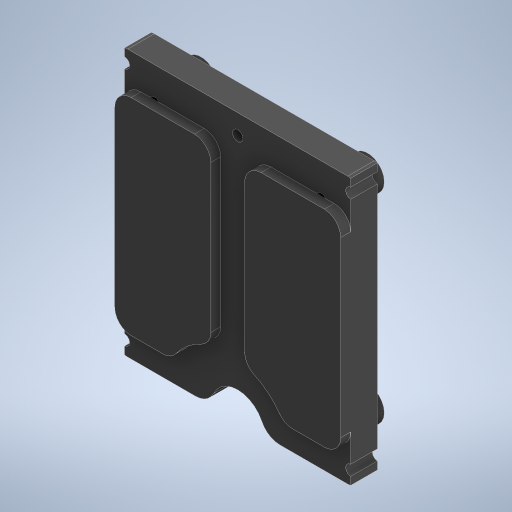
# Autodesk Inventor part: board_cover_inside
Saved by Autodesk Inventor 2024.1 (Build 281209000, 209)
## iProperties
Created: 2024-02-15
Part Number: board_cover_inside
Material: 一般
Document SubType Name: Modeling
Designer: hibik
Density: 1 g/cm^3
Appearance: 既定
Author: hibik
Autodesk Inventor part; units mm, degrees
ref_plane "YZ Plane" through (0, 0, 0) normal (1, 0, 0) x (0, 1, 0)
ref_plane "XZ Plane" through (0, 0, 0) normal (0, 1, 0) x (-1, 0, 0)
ref_plane "XY Plane" through (0, 0, 0) normal (0, 0, 1) x (1, 0, 0)
sketch "スケッチ1" plane through (0, 0, 0) normal (0, 0, 1) x (1, 0, 0)
  line L0 (18.5, 20) -> (-18.5, 20)
  line L1 (-18.5, 20) -> (-18.5, -20)
  line L2 (-18.5, -20) -> (18.5, -20)
  line L3 (18.5, -20) -> (18.5, 20)
  line L4 (18.5, 20) -> (-18.5, -20) construction
  line L5 (-18.5, 20) -> (18.5, -20) construction
  point P0 (0, 0)
  dimension "d0" = 37
  dimension "d1" = 40
  constraints: 12 end point, 2 midpoint, 2 parallel, 1 horizontal, 1 perpendicular
  measures "d0" distance of L2.end L1.end
  measures "d1" distance of L1.end L0.end
extrude "押し出し1" add sketch "スケッチ1" along normal blind 4
sketch "スケッチ3" plane through (0, 0, 4) normal (0, 0, 1) x (1, 0, 0)
  arc A0 (-6.3246, -20) -> (-3.614, -18.2857) centre (-6.3246, -17) ccw projected
  arc A1 (3.614, -18.2857) -> (-3.614, -18.2857) centre (0, -20) ccw projected
  arc A2 (3.614, -18.2857) -> (6.3246, -20) centre (6.3246, -17) ccw projected
  line L0 (19, -20) -> (6.3246, -20) projected
  line L1 (19, -20) -> (19, 20) projected
  line L2 (-19, 20) -> (19, 20) projected
  line L3 (-19, 20) -> (-19, -20) projected
  line L4 (-6.3246, -20) -> (-19, -20) projected
  line L5 (2, -9.0913) -> (2, 13) projected
  arc A3 (5, 16) -> (2, 13) centre (5, 13) ccw projected
  line L6 (5, 16) -> (14.5, 16) projected
  arc A4 (17.5, 13) -> (14.5, 16) centre (14.5, 13) ccw projected
  line L7 (17.5, 13) -> (17.5, -13) projected
  arc A5 (14.5, -16) -> (17.5, -13) centre (14.5, -13) ccw projected
  line L8 (14.5, -16) -> (9.7468, -16) projected
  arc A6 (7.3101, -14.75) -> (9.7468, -16) centre (9.7468, -13) ccw projected
  arc A7 (7.3101, -14.75) -> (3.75, -11.8185) centre (0, -20) ccw projected
  arc A8 (2, -9.0913) -> (3.75, -11.8185) centre (5, -9.0913) ccw projected
  arc A9 (-3.75, -11.8185) -> (-7.3101, -14.75) centre (0, -20) ccw projected
  arc A10 (-9.7468, -16) -> (-7.3101, -14.75) centre (-9.7468, -13) ccw projected
  line L9 (-9.7468, -16) -> (-14.5, -16) projected
  arc A11 (-17.5, -13) -> (-14.5, -16) centre (-14.5, -13) ccw projected
  line L10 (-17.5, -13) -> (-17.5, 13) projected
  arc A12 (-14.5, 16) -> (-17.5, 13) centre (-14.5, 13) ccw projected
  line L11 (-14.5, 16) -> (-5, 16) projected
  arc A13 (-2, 13) -> (-5, 16) centre (-5, 13) ccw projected
  line L12 (-2, 13) -> (-2, -9.0913) projected
  arc A14 (-3.75, -11.8185) -> (-2, -9.0913) centre (-5, -9.0913) ccw projected
  circle A15 centre (-17, -18) radius 0.8 projected
  circle A16 centre (-17, 18) radius 0.8 projected
  circle A17 centre (0, 17) radius 0.8 projected
  circle A18 centre (17, 18) radius 0.8 projected
  circle A19 centre (17, -18) radius 0.8 projected
  point P0 (0, 0)
extrude "押し出し3" add sketch "スケッチ3" along normal blind 1.5 draft -20 contours L5 A3 L6 A4 L7 A5 L8 A6 A7 A8 | A9 A10 L9 A11 L10 A12 L11 A13 L12 A14
fillet "フィレット1" radius 2 4 edges at (-18.5, 20, 2) (18.5, 20, 2) (18.5, -20, 2) (-18.5, -20, 2)
sketch "スケッチ4" plane through (0, 0, 4) normal (0, 0, 1) x (1, 0, 0)
  arc A0 (-6.3246, -20) -> (-3.614, -18.2857) centre (-6.3246, -17) ccw projected
  arc A1 (3.614, -18.2857) -> (-3.614, -18.2857) centre (0, -20) ccw projected
  arc A2 (3.614, -18.2857) -> (6.3246, -20) centre (6.3246, -17) ccw projected
  line L0 (19, -20) -> (6.3246, -20) projected
  line L1 (19, -20) -> (19, 20) projected
  line L2 (-19, 20) -> (19, 20) projected
  line L3 (-19, 20) -> (-19, -20) projected
  line L4 (-6.3246, -20) -> (-19, -20) projected
  line L5 (2, -9.0913) -> (2, 13) projected
  arc A3 (5, 16) -> (2, 13) centre (5, 13) ccw projected
  line L6 (5, 16) -> (14.5, 16) projected
  arc A4 (17.5, 13) -> (14.5, 16) centre (14.5, 13) ccw projected
  line L7 (17.5, 13) -> (17.5, -13) projected
  arc A5 (14.5, -16) -> (17.5, -13) centre (14.5, -13) ccw projected
  line L8 (14.5, -16) -> (9.7468, -16) projected
  arc A6 (7.3101, -14.75) -> (9.7468, -16) centre (9.7468, -13) ccw projected
  arc A7 (7.3101, -14.75) -> (3.75, -11.8185) centre (0, -20) ccw projected
  arc A8 (2, -9.0913) -> (3.75, -11.8185) centre (5, -9.0913) ccw projected
  arc A9 (-3.75, -11.8185) -> (-7.3101, -14.75) centre (0, -20) ccw projected
  arc A10 (-9.7468, -16) -> (-7.3101, -14.75) centre (-9.7468, -13) ccw projected
  line L9 (-9.7468, -16) -> (-14.5, -16) projected
  arc A11 (-17.5, -13) -> (-14.5, -16) centre (-14.5, -13) ccw projected
  line L10 (-17.5, -13) -> (-17.5, 13) projected
  arc A12 (-14.5, 16) -> (-17.5, 13) centre (-14.5, 13) ccw projected
  line L11 (-14.5, 16) -> (-5, 16) projected
  arc A13 (-2, 13) -> (-5, 16) centre (-5, 13) ccw projected
  line L12 (-2, 13) -> (-2, -9.0913) projected
  arc A14 (-3.75, -11.8185) -> (-2, -9.0913) centre (-5, -9.0913) ccw projected
  line L13 (14.5, -16) -> (9.7468, -16) projected
  arc A15 (7.3101, -14.75) -> (9.7468, -16) centre (9.7468, -13) ccw projected
  arc A16 (7.3101, -14.75) -> (3.75, -11.8185) centre (0, -20) ccw projected
  arc A17 (2, -9.0913) -> (3.75, -11.8185) centre (5, -9.0913) ccw projected
  line L14 (2, -9.0913) -> (2, 13) projected
  arc A18 (5, 16) -> (2, 13) centre (5, 13) ccw projected
  line L15 (5, 16) -> (14.5, 16) projected
  arc A19 (17.5, 13) -> (14.5, 16) centre (14.5, 13) ccw projected
  line L16 (17.5, 13) -> (17.5, -13) projected
  arc A20 (14.5, -16) -> (17.5, -13) centre (14.5, -13) ccw projected
  line L17 (-14.5, 16) -> (-5, 16) projected
  arc A21 (-2, 13) -> (-5, 16) centre (-5, 13) ccw projected
  line L18 (-2, 13) -> (-2, -9.0913) projected
  arc A22 (-3.75, -11.8185) -> (-2, -9.0913) centre (-5, -9.0913) ccw projected
  arc A23 (-3.75, -11.8185) -> (-7.3101, -14.75) centre (0, -20) ccw projected
  arc A24 (-9.7468, -16) -> (-7.3101, -14.75) centre (-9.7468, -13) ccw projected
  line L19 (-9.7468, -16) -> (-14.5, -16) projected
  arc A25 (-17.5, -13) -> (-14.5, -16) centre (-14.5, -13) ccw projected
  line L20 (-17.5, -13) -> (-17.5, 13) projected
  arc A26 (-14.5, 16) -> (-17.5, 13) centre (-14.5, 13) ccw projected
  arc A27 (-18.5, -18) -> (-16.5, -20) centre (-16.5, -18) ccw projected
  line L21 (-16.5, -20) -> (16.5, -20) projected
  arc A28 (16.5, -20) -> (18.5, -18) centre (16.5, -18) ccw projected
  line L22 (18.5, -18) -> (18.5, 18) projected
  arc A29 (18.5, 18) -> (16.5, 20) centre (16.5, 18) ccw projected
  line L23 (16.5, 20) -> (-16.5, 20) projected
  arc A30 (-16.5, 20) -> (-18.5, 18) centre (-16.5, 18) ccw projected
  line L24 (-18.5, 18) -> (-18.5, -18) projected
  circle A31 centre (-17, -18) radius 0.8 projected
  circle A32 centre (-17, 18) radius 0.8 projected
  circle A33 centre (0, 17) radius 0.8 projected
  circle A34 centre (17, 18) radius 0.8 projected
  circle A35 centre (17, -18) radius 0.8 projected
  point P0 (0, 0)
  point P1 (-6.3246, -20)
extrude "押し出し4" cut sketch "スケッチ4" against normal through all contours A0 A1 A2 L21
sketch "スケッチ5" plane through (0, 0, 0) normal (0, 0, -1) x (-1, 0, 0)
  circle A0 centre (17, -18) radius 0.8 projected
  circle A1 centre (17, 18) radius 0.8 projected
  circle A2 centre (0, 17) radius 0.8 projected
  circle A3 centre (-17, 18) radius 0.8 projected
  circle A4 centre (-17, -18) radius 0.8 projected
  arc A5 (3.614, -18.2857) -> (6.3246, -20) centre (6.3246, -17) ccw projected
  arc A6 (3.614, -18.2857) -> (-3.614, -18.2857) centre (0, -20) ccw projected
  arc A7 (-6.3246, -20) -> (-3.614, -18.2857) centre (-6.3246, -17) ccw projected
  line L0 (-19, -20) -> (-6.3246, -20) projected
  line L1 (-19, -20) -> (-19, 20) projected
  line L2 (19, 20) -> (-19, 20) projected
  line L3 (19, 20) -> (19, -20) projected
  line L4 (6.3246, -20) -> (19, -20) projected
  line L5 (-2, -9.0913) -> (-2, 13) projected
  arc A8 (-2, 13) -> (-5, 16) centre (-5, 13) ccw projected
  line L6 (-5, 16) -> (-14.5, 16) projected
  arc A9 (-14.5, 16) -> (-17.5, 13) centre (-14.5, 13) ccw projected
  line L7 (-17.5, 13) -> (-17.5, -13) projected
  arc A10 (-17.5, -13) -> (-14.5, -16) centre (-14.5, -13) ccw projected
  line L8 (-14.5, -16) -> (-9.7468, -16) projected
  arc A11 (-9.7468, -16) -> (-7.3101, -14.75) centre (-9.7468, -13) ccw projected
  arc A12 (-3.75, -11.8185) -> (-7.3101, -14.75) centre (0, -20) ccw projected
  arc A13 (-3.75, -11.8185) -> (-2, -9.0913) centre (-5, -9.0913) ccw projected
  arc A14 (7.3101, -14.75) -> (3.75, -11.8185) centre (0, -20) ccw projected
  arc A15 (7.3101, -14.75) -> (9.7468, -16) centre (9.7468, -13) ccw projected
  line L9 (9.7468, -16) -> (14.5, -16) projected
  arc A16 (14.5, -16) -> (17.5, -13) centre (14.5, -13) ccw projected
  line L10 (17.5, -13) -> (17.5, 13) projected
  arc A17 (17.5, 13) -> (14.5, 16) centre (14.5, 13) ccw projected
  line L11 (14.5, 16) -> (5, 16) projected
  arc A18 (5, 16) -> (2, 13) centre (5, 13) ccw projected
  line L12 (2, 13) -> (2, -9.0913) projected
  arc A19 (2, -9.0913) -> (3.75, -11.8185) centre (5, -9.0913) ccw projected
  point P0 (0, 0)
extrude "押し出し5" cut sketch "スケッチ5" against normal through all contours A0 | A1 | A2 | A3 | A4
sketch "スケッチ6" plane through (0, 0, 0) normal (0, 0, -1) x (-1, 0, 0)
  line L0 (-12.5, 15) -> (12.5, 15) construction
  line L1 (12.5, 15) -> (12.5, -15) construction
  line L2 (12.5, -15) -> (-12.5, -15) construction
  line L3 (-12.5, -15) -> (-12.5, 15) construction
  line L4 (-12.5, 15) -> (12.5, -15) construction
  line L5 (12.5, 15) -> (-12.5, -15) construction
  circle A0 centre (-12.5, 15) radius 0.8
  circle A1 centre (12.5, 15) radius 0.8
  circle A2 centre (-12.5, -15) radius 0.8
  circle A3 centre (12.5, -15) radius 0.8
  point P0 (0, 0)
  dimension "d19" = 25
  dimension "d20" = 30
  dimension "d21" = 1.6
  dimension "d22" = 1.6
  dimension "d23" = 1.6
  dimension "d24" = 1.6
  constraints: 12 end point, 4 centre point, 4 coincident, 2 midpoint, 2 parallel, 1 horizontal, 1 perpendicular
  measures "d19" distance of L0.start L0.end
  measures "d20" distance of L0.end L1.end
  measures "d21" diameter of A0
  measures "d22" diameter of A1
  measures "d23" diameter of A2
  measures "d24" diameter of A3
extrude "押し出し6" cut sketch "スケッチ6" against normal blind 4
sketch "スケッチ7" plane through (0, 0, 5.5) normal (0, 0, 1) x (1, 0, 0)
  line L0 (-14.5, 15.454) -> (-5, 15.454) projected
  arc A0 (-14.5, 15.454) -> (-16.954, 13) centre (-14.5, 13) ccw projected
  line L1 (-16.954, -13) -> (-16.954, 13) projected
  arc A1 (-16.954, -13) -> (-14.5, -15.454) centre (-14.5, -13) ccw projected
  line L2 (-9.7468, -15.454) -> (-14.5, -15.454) projected
  arc A2 (-9.7468, -15.454) -> (-7.7535, -14.4315) centre (-9.7468, -13) ccw projected
  arc A3 (-3.9775, -11.3222) -> (-7.7535, -14.4315) centre (0, -20) ccw projected
  arc A4 (-3.9775, -11.3222) -> (-2.546, -9.0913) centre (-5, -9.0913) ccw projected
  line L3 (-2.546, 13) -> (-2.546, -9.0913) projected
  arc A5 (-2.546, 13) -> (-5, 15.454) centre (-5, 13) ccw projected
  line L4 (14.5, -15.454) -> (9.7468, -15.454) projected
  arc A6 (14.5, -15.454) -> (16.954, -13) centre (14.5, -13) ccw projected
  line L5 (16.954, 13) -> (16.954, -13) projected
  arc A7 (16.954, 13) -> (14.5, 15.454) centre (14.5, 13) ccw projected
  line L6 (5, 15.454) -> (14.5, 15.454) projected
  arc A8 (5, 15.454) -> (2.546, 13) centre (5, 13) ccw projected
  line L7 (2.546, -9.0913) -> (2.546, 13) projected
  arc A9 (2.546, -9.0913) -> (3.9775, -11.3222) centre (5, -9.0913) ccw projected
  arc A10 (7.7535, -14.4315) -> (3.9775, -11.3222) centre (0, -20) ccw projected
  arc A11 (7.7535, -14.4315) -> (9.7468, -15.454) centre (9.7468, -13) ccw projected
  circle A12 centre (-17, 18) radius 0.8 projected
  circle A13 centre (-17, -18) radius 0.8 projected
  circle A14 centre (0, 17) radius 0.8 projected
  circle A15 centre (17, -18) radius 0.8 projected
  circle A16 centre (17, 18) radius 0.8 projected
  arc A17 (3.614, -18.2857) -> (6.3246, -20) centre (6.3246, -17) ccw projected
  line L8 (6.3246, -20) -> (16.5, -20) projected
  arc A18 (16.5, -20) -> (18.5, -18) centre (16.5, -18) ccw projected
  line L9 (18.5, -18) -> (18.5, 18) projected
  arc A19 (18.5, 18) -> (16.5, 20) centre (16.5, 18) ccw projected
  line L10 (16.5, 20) -> (-16.5, 20) projected
  arc A20 (-16.5, 20) -> (-18.5, 18) centre (-16.5, 18) ccw projected
  line L11 (-18.5, 18) -> (-18.5, -18) projected
  arc A21 (-18.5, -18) -> (-16.5, -20) centre (-16.5, -18) ccw projected
  line L12 (-16.5, -20) -> (-6.3246, -20) projected
  arc A22 (-6.3246, -20) -> (-3.614, -18.2857) centre (-6.3246, -17) ccw projected
  arc A23 (3.614, -18.2857) -> (-3.614, -18.2857) centre (0, -20) ccw projected
  line L13 (14.5, -16) -> (9.7468, -16) projected
  arc A24 (7.3101, -14.75) -> (9.7468, -16) centre (9.7468, -13) ccw projected
  arc A25 (7.3101, -14.75) -> (3.75, -11.8185) centre (0, -20) ccw projected
  arc A26 (2, -9.0913) -> (3.75, -11.8185) centre (5, -9.0913) ccw projected
  line L14 (2, -9.0913) -> (2, 13) projected
  arc A27 (5, 16) -> (2, 13) centre (5, 13) ccw projected
  line L15 (5, 16) -> (14.5, 16) projected
  arc A28 (17.5, 13) -> (14.5, 16) centre (14.5, 13) ccw projected
  line L16 (17.5, 13) -> (17.5, -13) projected
  arc A29 (14.5, -16) -> (17.5, -13) centre (14.5, -13) ccw projected
  line L17 (-14.5, 16) -> (-5, 16) projected
  arc A30 (-2, 13) -> (-5, 16) centre (-5, 13) ccw projected
  line L18 (-2, 13) -> (-2, -9.0913) projected
  arc A31 (-3.75, -11.8185) -> (-2, -9.0913) centre (-5, -9.0913) ccw projected
  arc A32 (-3.75, -11.8185) -> (-7.3101, -14.75) centre (0, -20) ccw projected
  arc A33 (-9.7468, -16) -> (-7.3101, -14.75) centre (-9.7468, -13) ccw projected
  line L19 (-9.7468, -16) -> (-14.5, -16) projected
  arc A34 (-17.5, -13) -> (-14.5, -16) centre (-14.5, -13) ccw projected
  line L20 (-17.5, -13) -> (-17.5, 13) projected
  arc A35 (-14.5, 16) -> (-17.5, 13) centre (-14.5, 13) ccw projected
  point P0 (0, 0)
extrude "押し出し7" cut sketch "スケッチ7" against normal up to surface (1.5 mm away) contours L13 A24 A25 A26 L14 A27 L15 A28 L16 A29 | L17 A30 L18 A31 A32 A33 L19 A34 L20 A35
sketch "スケッチ8" plane through (0, 0, 4) normal (0, 0, 1) x (1, 0, 0)
  line L0 (30, -20) -> (-30, -20)
  line L1 (-30, -20) -> (-30, 20)
  line L2 (-30, 20) -> (30, 20)
  line L3 (30, 20) -> (30, -20)
  line L4 (-16.954, 20) -> (16.954, 20)
  line L5 (16.954, 20) -> (16.954, -20)
  line L6 (16.954, -20) -> (-16.954, -20)
  line L7 (-16.954, -20) -> (-16.954, 20)
  line L8 (-16.954, -13) -> (-16.954, 13) projected
  line L9 (16.954, 13) -> (16.954, -13) projected
  line L10 (16.5, 20) -> (-16.5, 20) projected
  line L11 (6.3246, -20) -> (16.5, -20) projected
  point P0 (0, 0)
  point P1 (-16.954, -20)
  constraints: 16 end point, 4 collinear, 4 parallel, 2 horizontal, 2 perpendicular, 1 point on line
extrude "押し出し8" cut sketch "スケッチ8" against normal through all contours L0 L5 L2 L3 | L0 L1 L2 L7
sketch "スケッチ9" plane through (0, 0, 0) normal (0, 0, -1) x (-1, 0, 0)
  circle A0 centre (-12.5, 15) radius 0.8 projected
  circle A1 centre (12.5, 15) radius 0.8 projected
  circle A2 centre (12.5, -15) radius 0.8 projected
  line L0 (-9.7468, -15.454) -> (-11.8413, -15.454) projected
  circle A3 centre (-12.5, -15) radius 0.8 projected
  circle A4 centre (-12.5, 15) radius 2.5
  circle A5 centre (12.5, 15) radius 2.5
  circle A6 centre (12.5, -15) radius 2.5
  circle A7 centre (-12.5, -15) radius 2.5
  point P0 (0, 0)
  dimension "d32" = 5
  dimension "d33" = 5
  dimension "d34" = 5
  dimension "d35" = 5
  constraints: 4 centre point, 4 coincident, 1 other
  measures "d32" diameter of A4
  measures "d33" diameter of A5
  measures "d34" diameter of A6
  measures "d35" diameter of A7
extrude "押し出し9" add sketch "スケッチ9" along normal blind 3
